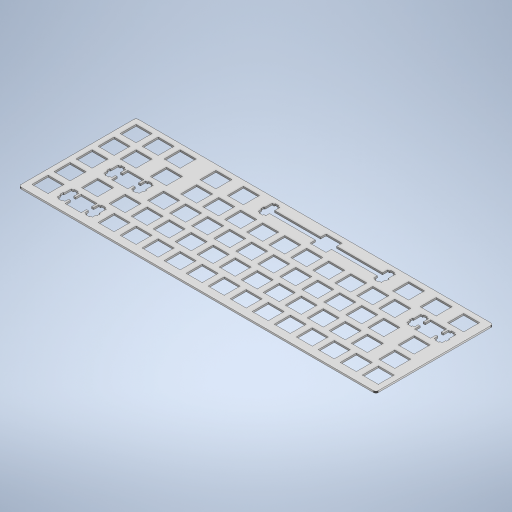
# Autodesk Inventor part: case_plate
Saved by Autodesk Inventor 2024 (Build 280153000, 153)
## iProperties
Created: 2023-08-02
Part Number: case_plate
Material: Generic
Document SubType Name: Modeling
Designer: Mika
Density: 1 g/cm^3
Appearance: Default
Author: Mika
Autodesk Inventor part; units mm, degrees
ref_plane "YZ Plane" through (0, 0, 0) normal (1, 0, 0) x (0, 1, 0)
ref_plane "XZ Plane" through (0, 0, 0) normal (0, 1, 0) x (-1, 0, 0)
ref_plane "XY Plane" through (0, 0, 0) normal (0, 0, 1) x (1, 0, 0)
sketch "Sketch1" plane through (0, 0, 0) normal (0, 1, 0) x (-1, 0, 0)
  line L0 (307.046, 101.8404) -> (307.202, 101.8337)
  line L1 (307.202, 101.8337) -> (307.359, 101.8157)
  line L2 (307.359, 101.8157) -> (307.512, 101.7853)
  line L3 (307.512, 101.7853) -> (307.665, 101.7426)
  line L4 (307.665, 101.7426) -> (307.811, 101.6876)
  line L5 (307.811, 101.6876) -> (307.953, 101.6227)
  line L6 (307.953, 101.6227) -> (308.091, 101.5458)
  line L7 (308.091, 101.5458) -> (308.222, 101.4587)
  line L8 (308.222, 101.4587) -> (308.344, 101.3609)
  line L9 (308.344, 101.3609) -> (308.46, 101.2548)
  line L10 (308.46, 101.2548) -> (308.566, 101.139)
  line L11 (308.566, 101.139) -> (308.664, 101.0166)
  line L12 (308.664, 101.0166) -> (308.751, 100.8854)
  line L13 (308.751, 100.8854) -> (308.828, 100.7478)
  line L14 (308.828, 100.7478) -> (308.894, 100.6056)
  line L15 (308.894, 100.6056) -> (308.948, 100.4596)
  line L16 (308.948, 100.4596) -> (308.991, 100.3068)
  line L17 (308.991, 100.3068) -> (309.021, 100.1537)
  line L18 (309.021, 100.1537) -> (309.039, 99.9967)
  line L19 (309.039, 99.9967) -> (309.047, 99.8398)
  line L20 (309.047, 99.8398) -> (309.047, 2.3399)
  line L21 (309.047, 2.3399) -> (309.039, 2.1842)
  line L22 (309.039, 2.1842) -> (309.021, 2.0271)
  line L23 (309.021, 2.0271) -> (308.991, 1.8741)
  line L24 (308.991, 1.8741) -> (308.948, 1.7212)
  line L25 (308.948, 1.7212) -> (308.894, 1.5751)
  line L26 (308.894, 1.5751) -> (308.828, 1.4332)
  line L27 (308.828, 1.4332) -> (308.751, 1.2954)
  line L28 (308.751, 1.2954) -> (308.664, 1.1644)
  line L29 (308.664, 1.1644) -> (308.566, 1.0418)
  line L30 (308.566, 1.0418) -> (308.46, 0.926)
  line L31 (308.46, 0.926) -> (308.344, 0.8199)
  line L32 (308.344, 0.8199) -> (308.222, 0.7221)
  line L33 (308.222, 0.7221) -> (308.091, 0.6353)
  line L34 (308.091, 0.6353) -> (307.953, 0.5581)
  line L35 (307.953, 0.5581) -> (307.811, 0.492)
  line L36 (307.811, 0.492) -> (307.665, 0.4382)
  line L37 (307.665, 0.4382) -> (307.512, 0.3955)
  line L38 (307.512, 0.3955) -> (307.359, 0.3652)
  line L39 (307.359, 0.3652) -> (307.202, 0.3473)
  line L40 (307.202, 0.3473) -> (307.045, 0.3404)
  line L41 (307.045, 0.3404) -> (2.096, 0.339)
  line L42 (2.096, 0.339) -> (1.9389, 0.3473)
  line L43 (1.9389, 0.3473) -> (1.7818, 0.3652)
  line L44 (1.7818, 0.3652) -> (1.6288, 0.3955)
  line L45 (1.6288, 0.3955) -> (1.4759, 0.4382)
  line L46 (1.4759, 0.4382) -> (1.3298, 0.492)
  line L47 (1.3298, 0.492) -> (1.1879, 0.5581)
  line L48 (1.1879, 0.5581) -> (1.0501, 0.6353)
  line L49 (1.0501, 0.6353) -> (0.9192, 0.7221)
  line L50 (0.9192, 0.7221) -> (0.7965, 0.8199)
  line L51 (0.7965, 0.8199) -> (0.6808, 0.926)
  line L52 (0.6808, 0.926) -> (0.5746, 1.0418)
  line L53 (0.5746, 1.0418) -> (0.4768, 1.1644)
  line L54 (0.4768, 1.1644) -> (0.39, 1.2954)
  line L55 (0.39, 1.2954) -> (0.3128, 1.4332)
  line L56 (0.3128, 1.4332) -> (0.248, 1.5751)
  line L57 (0.248, 1.5751) -> (0.1929, 1.7212)
  line L58 (0.1929, 1.7212) -> (0.1502, 1.8741)
  line L59 (0.1502, 1.8741) -> (0.1199, 2.0271)
  line L60 (0.1199, 2.0271) -> (0.102, 2.1842)
  line L61 (0.102, 2.1842) -> (0.0951, 2.3399)
  line L62 (0.0951, 2.3399) -> (0.0951, 99.8384)
  line L63 (0.0951, 99.8384) -> (0.102, 99.9953)
  line L64 (0.102, 99.9953) -> (0.1199, 100.1523)
  line L65 (0.1199, 100.1523) -> (0.1502, 100.3054)
  line L66 (0.1502, 100.3054) -> (0.1929, 100.4582)
  line L67 (0.1929, 100.4582) -> (0.248, 100.6042)
  line L68 (0.248, 100.6042) -> (0.3128, 100.7464)
  line L69 (0.3128, 100.7464) -> (0.39, 100.884)
  line L70 (0.39, 100.884) -> (0.4768, 101.0152)
  line L71 (0.4768, 101.0152) -> (0.5746, 101.1376)
  line L72 (0.5746, 101.1376) -> (0.6807, 101.2534)
  line L73 (0.6807, 101.2534) -> (0.7965, 101.3595)
  line L74 (0.7965, 101.3595) -> (0.9191, 101.4573)
  line L75 (0.9191, 101.4573) -> (1.0501, 101.5444)
  line L76 (1.0501, 101.5444) -> (1.1879, 101.6213)
  line L77 (1.1879, 101.6213) -> (1.3298, 101.6862)
  line L78 (1.3298, 101.6862) -> (1.4759, 101.7412)
  line L79 (1.4759, 101.7412) -> (1.6288, 101.7839)
  line L80 (1.6288, 101.7839) -> (1.7818, 101.8143)
  line L81 (1.7818, 101.8143) -> (1.9389, 101.8323)
  line L82 (1.9389, 101.8323) -> (2.096, 101.839)
  line L83 (2.096, 101.839) -> (307.046, 101.8404)
  line L84 (126.213, 18.8654) -> (126.213, 14.1663)
  line L85 (126.213, 14.1663) -> (86.4387, 14.1663)
  line L86 (86.4387, 14.1663) -> (86.4387, 17.395)
  line L87 (86.4387, 17.395) -> (84.7136, 17.395)
  line L88 (84.7136, 17.395) -> (84.7136, 18.3155)
  line L89 (84.7136, 18.3155) -> (81.5633, 18.3155)
  line L90 (81.5633, 18.3155) -> (81.5633, 17.395)
  line L91 (81.5633, 17.395) -> (79.8382, 17.395)
  line L92 (79.8382, 17.395) -> (79.8382, 14.1663)
  line L93 (79.8382, 14.1663) -> (79.0141, 14.1663)
  line L94 (79.0141, 14.1663) -> (79.0141, 11.5163)
  line L95 (79.0141, 11.5163) -> (79.8382, 11.5163)
  line L96 (79.8382, 11.5163) -> (79.8382, 5.2462)
  line L97 (79.8382, 5.2462) -> (81.5633, 5.2462)
  line L98 (81.5633, 5.2462) -> (81.5633, 4.265)
  line L99 (81.5633, 4.265) -> (84.7136, 4.265)
  line L100 (84.7136, 4.265) -> (84.7136, 5.2462)
  line L101 (84.7136, 5.2462) -> (86.4387, 5.2462)
  line L102 (86.4387, 5.2462) -> (86.4387, 9.7166)
  line L103 (86.4387, 9.7166) -> (126.213, 9.7166)
  line L104 (126.213, 9.7166) -> (126.213, 5.0161)
  line L105 (126.213, 5.0161) -> (140.064, 5.0161)
  line L106 (140.064, 5.0161) -> (140.064, 9.7166)
  line L107 (140.064, 9.7166) -> (179.838, 9.7166)
  line L108 (179.838, 9.7166) -> (179.838, 5.2462)
  line L109 (179.838, 5.2462) -> (181.563, 5.2462)
  line L110 (181.563, 5.2462) -> (181.563, 4.265)
  line L111 (181.563, 4.265) -> (184.714, 4.265)
  line L112 (184.714, 4.265) -> (184.714, 5.2462)
  line L113 (184.714, 5.2462) -> (186.439, 5.2462)
  line L114 (186.439, 5.2462) -> (186.439, 11.5163)
  line L115 (186.439, 11.5163) -> (187.263, 11.5163)
  line L116 (187.263, 11.5163) -> (187.263, 14.1663)
  line L117 (187.263, 14.1663) -> (186.439, 14.1663)
  line L118 (186.439, 14.1663) -> (186.439, 17.395)
  line L119 (186.439, 17.395) -> (184.714, 17.395)
  line L120 (184.714, 17.395) -> (184.714, 18.3155)
  line L121 (184.714, 18.3155) -> (181.563, 18.3155)
  line L122 (181.563, 18.3155) -> (181.563, 17.395)
  line L123 (181.563, 17.395) -> (179.838, 17.395)
  line L124 (179.838, 17.395) -> (179.838, 14.1663)
  line L125 (179.838, 14.1663) -> (140.064, 14.1663)
  line L126 (140.064, 14.1663) -> (140.064, 18.8654)
  line L127 (140.064, 18.8654) -> (126.213, 18.8654)
  line L128 (7.152, 18.8654) -> (21.0013, 18.8654)
  line L129 (21.0013, 18.8654) -> (21.0013, 5.0161)
  line L130 (21.0013, 5.0161) -> (7.152, 5.0161)
  line L131 (7.152, 5.0161) -> (7.152, 18.8654)
  line L132 (30.9631, 18.8654) -> (44.8137, 18.8654)
  line L133 (44.8137, 18.8654) -> (44.8137, 5.0161)
  line L134 (44.8137, 5.0161) -> (30.9631, 5.0161)
  line L135 (30.9631, 5.0161) -> (30.9631, 18.8654)
  line L136 (54.7769, 18.8654) -> (68.6262, 18.8654)
  line L137 (68.6262, 18.8654) -> (68.6262, 5.0161)
  line L138 (68.6262, 5.0161) -> (54.7769, 5.0161)
  line L139 (54.7769, 5.0161) -> (54.7769, 18.8654)
  line L140 (197.652, 18.8654) -> (211.501, 18.8654)
  line L141 (211.501, 18.8654) -> (211.501, 5.0161)
  line L142 (211.501, 5.0161) -> (197.652, 5.0161)
  line L143 (197.652, 5.0161) -> (197.652, 18.8654)
  line L144 (221.463, 18.8654) -> (235.314, 18.8654)
  line L145 (235.314, 18.8654) -> (235.314, 5.0161)
  line L146 (235.314, 5.0161) -> (221.463, 5.0161)
  line L147 (221.463, 5.0161) -> (221.463, 18.8654)
  line L148 (252.421, 18.8654) -> (266.27, 18.8654)
  line L149 (266.27, 18.8654) -> (266.27, 5.0161)
  line L150 (266.27, 5.0161) -> (252.421, 5.0161)
  line L151 (252.421, 5.0161) -> (252.421, 18.8654)
  line L152 (271.471, 18.8654) -> (285.32, 18.8654)
  line L153 (285.32, 18.8654) -> (285.32, 5.0161)
  line L154 (285.32, 5.0161) -> (271.471, 5.0161)
  line L155 (271.471, 5.0161) -> (271.471, 18.8654)
  line L156 (290.521, 18.8654) -> (304.37, 18.8654)
  line L157 (304.37, 18.8654) -> (304.37, 5.0161)
  line L158 (304.37, 5.0161) -> (290.521, 5.0161)
  line L159 (290.521, 5.0161) -> (290.521, 18.8654)
  line L160 (16.677, 37.9155) -> (16.677, 33.2163)
  line L161 (16.677, 33.2163) -> (15.0013, 33.2163)
  line L162 (15.0013, 33.2163) -> (15.0013, 36.4451)
  line L163 (15.0013, 36.4451) -> (13.276, 36.4451)
  line L164 (13.276, 36.4451) -> (13.276, 37.3655)
  line L165 (13.276, 37.3655) -> (10.1258, 37.3655)
  line L166 (10.1258, 37.3655) -> (10.1258, 36.4451)
  line L167 (10.1258, 36.4451) -> (8.4019, 36.4451)
  line L168 (8.4019, 36.4451) -> (8.4019, 33.2163)
  line L169 (8.4019, 33.2163) -> (7.5765, 33.2163)
  line L170 (7.5765, 33.2163) -> (7.5765, 30.5663)
  line L171 (7.5765, 30.5663) -> (8.4019, 30.5663)
  line L172 (8.4019, 30.5663) -> (8.4019, 24.2962)
  line L173 (8.4019, 24.2962) -> (10.1258, 24.2962)
  line L174 (10.1258, 24.2962) -> (10.1258, 23.315)
  line L175 (10.1258, 23.315) -> (13.276, 23.315)
  line L176 (13.276, 23.315) -> (13.276, 24.2962)
  line L177 (13.276, 24.2962) -> (15.0013, 24.2962)
  line L178 (15.0013, 24.2962) -> (15.0013, 28.7652)
  line L179 (15.0013, 28.7652) -> (16.677, 28.7652)
  line L180 (16.677, 28.7652) -> (16.677, 24.0661)
  line L181 (16.677, 24.0661) -> (30.5263, 24.0661)
  line L182 (30.5263, 24.0661) -> (30.5263, 28.7652)
  line L183 (30.5263, 28.7652) -> (32.202, 28.7652)
  line L184 (32.202, 28.7652) -> (32.202, 24.2962)
  line L185 (32.202, 24.2962) -> (33.9259, 24.2962)
  line L186 (33.9259, 24.2962) -> (33.9259, 23.315)
  line L187 (33.9259, 23.315) -> (37.0762, 23.315)
  line L188 (37.0762, 23.315) -> (37.0762, 24.2962)
  line L189 (37.0762, 24.2962) -> (38.8013, 24.2962)
  line L190 (38.8013, 24.2962) -> (38.8013, 30.5663)
  line L191 (38.8013, 30.5663) -> (39.6268, 30.5663)
  line L192 (39.6268, 30.5663) -> (39.6268, 33.2163)
  line L193 (39.6268, 33.2163) -> (38.8013, 33.2163)
  line L194 (38.8013, 33.2163) -> (38.8013, 36.4451)
  line L195 (38.8013, 36.4451) -> (37.0762, 36.4451)
  line L196 (37.0762, 36.4451) -> (37.0762, 37.3655)
  line L197 (37.0762, 37.3655) -> (33.9259, 37.3655)
  line L198 (33.9259, 37.3655) -> (33.9259, 36.4451)
  line L199 (33.9259, 36.4451) -> (32.202, 36.4451)
  line L200 (32.202, 36.4451) -> (32.202, 33.2163)
  line L201 (32.202, 33.2163) -> (30.5263, 33.2163)
  line L202 (30.5263, 33.2163) -> (30.5263, 37.9155)
  line L203 (30.5263, 37.9155) -> (16.677, 37.9155)
  line L204 (47.6321, 37.9155) -> (61.4825, 37.9155)
  line L205 (61.4825, 37.9155) -> (61.4825, 24.0661)
  line L206 (61.4825, 24.0661) -> (47.6321, 24.0661)
  line L207 (47.6321, 24.0661) -> (47.6321, 37.9155)
  line L208 (66.6821, 37.9155) -> (80.5325, 37.9155)
  line L209 (80.5325, 37.9155) -> (80.5325, 24.0661)
  line L210 (80.5325, 24.0661) -> (66.6821, 24.0661)
  line L211 (66.6821, 24.0661) -> (66.6821, 37.9155)
  line L212 (85.7321, 37.9155) -> (99.5825, 37.9155)
  line L213 (99.5825, 37.9155) -> (99.5825, 24.0661)
  line L214 (99.5825, 24.0661) -> (85.7321, 24.0661)
  line L215 (85.7321, 24.0661) -> (85.7321, 37.9155)
  line L216 (104.782, 37.9155) -> (118.632, 37.9155)
  line L217 (118.632, 37.9155) -> (118.632, 24.0661)
  line L218 (118.632, 24.0661) -> (104.782, 24.0661)
  line L219 (104.782, 24.0661) -> (104.782, 37.9155)
  line L220 (123.832, 37.9155) -> (137.682, 37.9155)
  line L221 (137.682, 37.9155) -> (137.682, 24.0661)
  line L222 (137.682, 24.0661) -> (123.832, 24.0661)
  line L223 (123.832, 24.0661) -> (123.832, 37.9155)
  line L224 (142.882, 37.9155) -> (156.732, 37.9155)
  line L225 (156.732, 37.9155) -> (156.732, 24.0661)
  line L226 (156.732, 24.0661) -> (142.882, 24.0661)
  line L227 (142.882, 24.0661) -> (142.882, 37.9155)
  line L228 (161.932, 37.9155) -> (175.782, 37.9155)
  line L229 (175.782, 37.9155) -> (175.782, 24.0661)
  line L230 (175.782, 24.0661) -> (161.932, 24.0661)
  line L231 (161.932, 24.0661) -> (161.932, 37.9155)
  line L232 (180.982, 37.9155) -> (194.832, 37.9155)
  line L233 (194.832, 37.9155) -> (194.832, 24.0661)
  line L234 (194.832, 24.0661) -> (180.982, 24.0661)
  line L235 (180.982, 24.0661) -> (180.982, 37.9155)
  line L236 (200.032, 37.9155) -> (213.882, 37.9155)
  line L237 (213.882, 37.9155) -> (213.882, 24.0661)
  line L238 (213.882, 24.0661) -> (200.032, 24.0661)
  line L239 (200.032, 24.0661) -> (200.032, 37.9155)
  line L240 (219.082, 37.9155) -> (232.932, 37.9155)
  line L241 (232.932, 37.9155) -> (232.932, 24.0661)
  line L242 (232.932, 24.0661) -> (219.082, 24.0661)
  line L243 (219.082, 24.0661) -> (219.082, 37.9155)
  line L244 (245.277, 37.9155) -> (259.126, 37.9155)
  line L245 (259.126, 37.9155) -> (259.126, 24.0661)
  line L246 (259.126, 24.0661) -> (245.277, 24.0661)
  line L247 (245.277, 24.0661) -> (245.277, 37.9155)
  line L248 (271.471, 37.9155) -> (285.32, 37.9155)
  line L249 (285.32, 37.9155) -> (285.32, 24.0661)
  line L250 (285.32, 24.0661) -> (271.471, 24.0661)
  line L251 (271.471, 24.0661) -> (271.471, 37.9155)
  line L252 (290.521, 37.9155) -> (304.37, 37.9155)
  line L253 (304.37, 37.9155) -> (304.37, 24.0661)
  line L254 (304.37, 24.0661) -> (290.521, 24.0661)
  line L255 (290.521, 24.0661) -> (290.521, 37.9155)
  line L256 (259.563, 56.9655) -> (259.563, 52.2661)
  line L257 (259.563, 52.2661) -> (257.889, 52.2661)
  line L258 (257.889, 52.2661) -> (257.889, 55.4951)
  line L259 (257.889, 55.4951) -> (256.162, 55.4951)
  line L260 (256.162, 55.4951) -> (256.162, 56.4155)
  line L261 (256.162, 56.4155) -> (253.013, 56.4155)
  line L262 (253.013, 56.4155) -> (253.013, 55.4951)
  line L263 (253.013, 55.4951) -> (251.288, 55.4951)
  line L264 (251.288, 55.4951) -> (251.288, 52.2661)
  line L265 (251.288, 52.2661) -> (250.464, 52.2661)
  line L266 (250.464, 52.2661) -> (250.464, 49.6164)
  line L267 (250.464, 49.6164) -> (251.288, 49.6164)
  line L268 (251.288, 49.6164) -> (251.288, 43.3462)
  line L269 (251.288, 43.3462) -> (253.013, 43.3462)
  line L270 (253.013, 43.3462) -> (253.013, 42.3651)
  line L271 (253.013, 42.3651) -> (256.162, 42.3651)
  line L272 (256.162, 42.3651) -> (256.162, 43.3462)
  line L273 (256.162, 43.3462) -> (257.889, 43.3462)
  line L274 (257.889, 43.3462) -> (257.889, 47.8151)
  line L275 (257.889, 47.8151) -> (259.563, 47.8151)
  line L276 (259.563, 47.8151) -> (259.563, 43.1161)
  line L277 (259.563, 43.1161) -> (273.414, 43.1161)
  line L278 (273.414, 43.1161) -> (273.414, 47.8151)
  line L279 (273.414, 47.8151) -> (275.088, 47.8151)
  line L280 (275.088, 47.8151) -> (275.088, 43.3462)
  line L281 (275.088, 43.3462) -> (276.813, 43.3462)
  line L282 (276.813, 43.3462) -> (276.813, 42.3651)
  line L283 (276.813, 42.3651) -> (279.964, 42.3651)
  line L284 (279.964, 42.3651) -> (279.964, 43.3462)
  line L285 (279.964, 43.3462) -> (281.689, 43.3462)
  line L286 (281.689, 43.3462) -> (281.689, 49.6164)
  line L287 (281.689, 49.6164) -> (282.513, 49.6164)
  line L288 (282.513, 49.6164) -> (282.513, 52.2661)
  line L289 (282.513, 52.2661) -> (281.689, 52.2661)
  line L290 (281.689, 52.2661) -> (281.689, 55.4951)
  line L291 (281.689, 55.4951) -> (279.964, 55.4951)
  line L292 (279.964, 55.4951) -> (279.964, 56.4155)
  line L293 (279.964, 56.4155) -> (276.813, 56.4155)
  line L294 (276.813, 56.4155) -> (276.813, 55.4951)
  line L295 (276.813, 55.4951) -> (275.088, 55.4951)
  line L296 (275.088, 55.4951) -> (275.088, 52.2661)
  line L297 (275.088, 52.2661) -> (273.414, 52.2661)
  line L298 (273.414, 52.2661) -> (273.414, 56.9655)
  line L299 (273.414, 56.9655) -> (259.563, 56.9655)
  line L300 (11.9131, 56.9655) -> (25.7638, 56.9655)
  line L301 (25.7638, 56.9655) -> (25.7638, 43.1161)
  line L302 (25.7638, 43.1161) -> (11.9131, 43.1161)
  line L303 (11.9131, 43.1161) -> (11.9131, 56.9655)
  line L304 (38.1071, 56.9655) -> (51.9575, 56.9655)
  line L305 (51.9575, 56.9655) -> (51.9575, 43.1161)
  line L306 (51.9575, 43.1161) -> (38.1071, 43.1161)
  line L307 (38.1071, 43.1161) -> (38.1071, 56.9655)
  line L308 (57.1571, 56.9655) -> (71.0075, 56.9655)
  line L309 (71.0075, 56.9655) -> (71.0075, 43.1161)
  line L310 (71.0075, 43.1161) -> (57.1571, 43.1161)
  line L311 (57.1571, 43.1161) -> (57.1571, 56.9655)
  line L312 (76.2071, 56.9655) -> (90.0575, 56.9655)
  line L313 (90.0575, 56.9655) -> (90.0575, 43.1161)
  line L314 (90.0575, 43.1161) -> (76.2071, 43.1161)
  line L315 (76.2071, 43.1161) -> (76.2071, 56.9655)
  line L316 (95.2571, 56.9655) -> (109.107, 56.9655)
  line L317 (109.107, 56.9655) -> (109.107, 43.1161)
  line L318 (109.107, 43.1161) -> (95.2571, 43.1161)
  line L319 (95.2571, 43.1161) -> (95.2571, 56.9655)
  line L320 (114.307, 56.9655) -> (128.157, 56.9655)
  line L321 (128.157, 56.9655) -> (128.157, 43.1161)
  line L322 (128.157, 43.1161) -> (114.307, 43.1161)
  line L323 (114.307, 43.1161) -> (114.307, 56.9655)
  line L324 (133.357, 56.9655) -> (147.207, 56.9655)
  line L325 (147.207, 56.9655) -> (147.207, 43.1161)
  line L326 (147.207, 43.1161) -> (133.357, 43.1161)
  line L327 (133.357, 43.1161) -> (133.357, 56.9655)
  line L328 (152.407, 56.9655) -> (166.257, 56.9655)
  line L329 (166.257, 56.9655) -> (166.257, 43.1161)
  line L330 (166.257, 43.1161) -> (152.407, 43.1161)
  line L331 (152.407, 43.1161) -> (152.407, 56.9655)
  line L332 (171.457, 56.9655) -> (185.307, 56.9655)
  line L333 (185.307, 56.9655) -> (185.307, 43.1161)
  line L334 (185.307, 43.1161) -> (171.457, 43.1161)
  line L335 (171.457, 43.1161) -> (171.457, 56.9655)
  line L336 (190.507, 56.9655) -> (204.357, 56.9655)
  line L337 (204.357, 56.9655) -> (204.357, 43.1161)
  line L338 (204.357, 43.1161) -> (190.507, 43.1161)
  line L339 (190.507, 43.1161) -> (190.507, 56.9655)
  line L340 (209.557, 56.9655) -> (223.407, 56.9655)
  line L341 (223.407, 56.9655) -> (223.407, 43.1161)
  line L342 (223.407, 43.1161) -> (209.557, 43.1161)
  line L343 (209.557, 43.1161) -> (209.557, 56.9655)
  line L344 (228.607, 56.9655) -> (242.457, 56.9655)
  line L345 (242.457, 56.9655) -> (242.457, 43.1161)
  line L346 (242.457, 43.1161) -> (228.607, 43.1161)
  line L347 (228.607, 43.1161) -> (228.607, 56.9655)
  line L348 (290.521, 56.9655) -> (304.37, 56.9655)
  line L349 (304.37, 56.9655) -> (304.37, 43.1161)
  line L350 (304.37, 43.1161) -> (290.521, 43.1161)
  line L351 (290.521, 43.1161) -> (290.521, 56.9655)
  line L352 (9.5319, 76.0155) -> (23.3826, 76.0155)
  line L353 (23.3826, 76.0155) -> (23.3826, 62.1661)
  line L354 (23.3826, 62.1661) -> (9.5319, 62.1661)
  line L355 (9.5319, 62.1661) -> (9.5319, 76.0155)
  line L356 (33.3458, 76.0155) -> (47.195, 76.0155)
  line L357 (47.195, 76.0155) -> (47.195, 62.1661)
  line L358 (47.195, 62.1661) -> (33.3458, 62.1661)
  line L359 (33.3458, 62.1661) -> (33.3458, 76.0155)
  line L360 (52.3956, 76.0155) -> (66.245, 76.0155)
  line L361 (66.245, 76.0155) -> (66.245, 62.1661)
  line L362 (66.245, 62.1661) -> (52.3956, 62.1661)
  line L363 (52.3956, 62.1661) -> (52.3956, 76.0155)
  line L364 (71.4456, 76.0155) -> (85.295, 76.0155)
  line L365 (85.295, 76.0155) -> (85.295, 62.1661)
  line L366 (85.295, 62.1661) -> (71.4456, 62.1661)
  line L367 (71.4456, 62.1661) -> (71.4456, 76.0155)
  line L368 (90.4946, 76.0155) -> (104.345, 76.0155)
  line L369 (104.345, 76.0155) -> (104.345, 62.1661)
  line L370 (104.345, 62.1661) -> (90.4946, 62.1661)
  line L371 (90.4946, 62.1661) -> (90.4946, 76.0155)
  line L372 (109.545, 76.0155) -> (123.395, 76.0155)
  line L373 (123.395, 76.0155) -> (123.395, 62.1661)
  line L374 (123.395, 62.1661) -> (109.545, 62.1661)
  line L375 (109.545, 62.1661) -> (109.545, 76.0155)
  line L376 (128.595, 76.0155) -> (142.445, 76.0155)
  line L377 (142.445, 76.0155) -> (142.445, 62.1661)
  line L378 (142.445, 62.1661) -> (128.595, 62.1661)
  line L379 (128.595, 62.1661) -> (128.595, 76.0155)
  line L380 (147.645, 76.0155) -> (161.495, 76.0155)
  line L381 (161.495, 76.0155) -> (161.495, 62.1661)
  line L382 (161.495, 62.1661) -> (147.645, 62.1661)
  line L383 (147.645, 62.1661) -> (147.645, 76.0155)
  line L384 (166.696, 76.0155) -> (180.545, 76.0155)
  line L385 (180.545, 76.0155) -> (180.545, 62.1661)
  line L386 (180.545, 62.1661) -> (166.696, 62.1661)
  line L387 (166.696, 62.1661) -> (166.696, 76.0155)
  line L388 (185.746, 76.0155) -> (199.595, 76.0155)
  line L389 (199.595, 76.0155) -> (199.595, 62.1661)
  line L390 (199.595, 62.1661) -> (185.746, 62.1661)
  line L391 (185.746, 62.1661) -> (185.746, 76.0155)
  line L392 (204.796, 76.0155) -> (218.645, 76.0155)
  line L393 (218.645, 76.0155) -> (218.645, 62.1661)
  line L394 (218.645, 62.1661) -> (204.796, 62.1661)
  line L395 (204.796, 62.1661) -> (204.796, 76.0155)
  line L396 (223.846, 76.0155) -> (237.695, 76.0155)
  line L397 (237.695, 76.0155) -> (237.695, 62.1661)
  line L398 (237.695, 62.1661) -> (223.846, 62.1661)
  line L399 (223.846, 62.1661) -> (223.846, 76.0155)
  line L400 (242.896, 76.0155) -> (256.745, 76.0155)
  line L401 (256.745, 76.0155) -> (256.745, 62.1661)
  line L402 (256.745, 62.1661) -> (242.896, 62.1661)
  line L403 (242.896, 62.1661) -> (242.896, 76.0155)
  line L404 (266.707, 76.0155) -> (280.557, 76.0155)
  line L405 (280.557, 76.0155) -> (280.557, 62.1661)
  line L406 (280.557, 62.1661) -> (266.707, 62.1661)
  line L407 (266.707, 62.1661) -> (266.707, 76.0155)
  line L408 (290.521, 76.0155) -> (304.37, 76.0155)
  line L409 (304.37, 76.0155) -> (304.37, 62.1661)
  line L410 (304.37, 62.1661) -> (290.521, 62.1661)
  line L411 (290.521, 62.1661) -> (290.521, 76.0155)
  line L412 (261.946, 95.0655) -> (261.946, 90.3661)
  line L413 (261.946, 90.3661) -> (260.27, 90.3661)
  line L414 (260.27, 90.3661) -> (260.27, 93.5951)
  line L415 (260.27, 93.5951) -> (258.546, 93.5951)
  line L416 (258.546, 93.5951) -> (258.546, 94.5155)
  line L417 (258.546, 94.5155) -> (255.396, 94.5155)
  line L418 (255.396, 94.5155) -> (255.396, 93.5951)
  line L419 (255.396, 93.5951) -> (253.67, 93.5951)
  line L420 (253.67, 93.5951) -> (253.67, 90.3661)
  line L421 (253.67, 90.3661) -> (252.845, 90.3661)
  line L422 (252.845, 90.3661) -> (252.845, 87.7164)
  line L423 (252.845, 87.7164) -> (253.67, 87.7164)
  line L424 (253.67, 87.7164) -> (253.67, 81.4462)
  line L425 (253.67, 81.4462) -> (255.396, 81.4462)
  line L426 (255.396, 81.4462) -> (255.396, 80.4651)
  line L427 (255.396, 80.4651) -> (258.546, 80.4651)
  line L428 (258.546, 80.4651) -> (258.546, 81.4462)
  line L429 (258.546, 81.4462) -> (260.27, 81.4462)
  line L430 (260.27, 81.4462) -> (260.27, 85.9151)
  line L431 (260.27, 85.9151) -> (261.946, 85.9151)
  line L432 (261.946, 85.9151) -> (261.946, 81.2161)
  line L433 (261.946, 81.2161) -> (275.795, 81.2161)
  line L434 (275.795, 81.2161) -> (275.795, 85.9151)
  line L435 (275.795, 85.9151) -> (277.471, 85.9151)
  line L436 (277.471, 85.9151) -> (277.471, 81.4462)
  line L437 (277.471, 81.4462) -> (279.196, 81.4462)
  line L438 (279.196, 81.4462) -> (279.196, 80.4651)
  line L439 (279.196, 80.4651) -> (282.345, 80.4651)
  line L440 (282.345, 80.4651) -> (282.345, 81.4462)
  line L441 (282.345, 81.4462) -> (284.07, 81.4462)
  line L442 (284.07, 81.4462) -> (284.07, 87.7164)
  line L443 (284.07, 87.7164) -> (284.896, 87.7164)
  line L444 (284.896, 87.7164) -> (284.896, 90.3661)
  line L445 (284.896, 90.3661) -> (284.07, 90.3661)
  line L446 (284.07, 90.3661) -> (284.07, 93.5951)
  line L447 (284.07, 93.5951) -> (282.345, 93.5951)
  line L448 (282.345, 93.5951) -> (282.345, 94.5155)
  line L449 (282.345, 94.5155) -> (279.196, 94.5155)
  line L450 (279.196, 94.5155) -> (279.196, 93.5951)
  line L451 (279.196, 93.5951) -> (277.471, 93.5951)
  line L452 (277.471, 93.5951) -> (277.471, 90.3661)
  line L453 (277.471, 90.3661) -> (275.795, 90.3661)
  line L454 (275.795, 90.3661) -> (275.795, 95.0655)
  line L455 (275.795, 95.0655) -> (261.946, 95.0655)
  line L456 (4.7708, 95.0655) -> (18.6201, 95.0655)
  line L457 (18.6201, 95.0655) -> (18.6201, 81.2161)
  line L458 (18.6201, 81.2161) -> (4.7708, 81.2161)
  line L459 (4.7708, 81.2161) -> (4.7708, 95.0655)
  line L460 (23.8208, 95.0655) -> (37.67, 95.0655)
  line L461 (37.67, 95.0655) -> (37.67, 81.2161)
  line L462 (37.67, 81.2161) -> (23.8208, 81.2161)
  line L463 (23.8208, 81.2161) -> (23.8208, 95.0655)
  line L464 (42.8706, 95.0655) -> (56.72, 95.0655)
  line L465 (56.72, 95.0655) -> (56.72, 81.2161)
  line L466 (56.72, 81.2161) -> (42.8706, 81.2161)
  line L467 (42.8706, 81.2161) -> (42.8706, 95.0655)
  line L468 (61.9206, 95.0655) -> (75.77, 95.0655)
  line L469 (75.77, 95.0655) -> (75.77, 81.2161)
  line L470 (75.77, 81.2161) -> (61.9206, 81.2161)
  line L471 (61.9206, 81.2161) -> (61.9206, 95.0655)
  line L472 (80.9706, 95.0655) -> (94.82, 95.0655)
  line L473 (94.82, 95.0655) -> (94.82, 81.2161)
  line L474 (94.82, 81.2161) -> (80.9706, 81.2161)
  line L475 (80.9706, 81.2161) -> (80.9706, 95.0655)
  line L476 (100.021, 95.0655) -> (113.87, 95.0655)
  line L477 (113.87, 95.0655) -> (113.87, 81.2161)
  line L478 (113.87, 81.2161) -> (100.021, 81.2161)
  line L479 (100.021, 81.2161) -> (100.021, 95.0655)
  line L480 (119.071, 95.0655) -> (132.92, 95.0655)
  line L481 (132.92, 95.0655) -> (132.92, 81.2161)
  line L482 (132.92, 81.2161) -> (119.071, 81.2161)
  line L483 (119.071, 81.2161) -> (119.071, 95.0655)
  line L484 (138.121, 95.0655) -> (151.97, 95.0655)
  line L485 (151.97, 95.0655) -> (151.97, 81.2161)
  line L486 (151.97, 81.2161) -> (138.121, 81.2161)
  line L487 (138.121, 81.2161) -> (138.121, 95.0655)
  line L488 (157.171, 95.0655) -> (171.02, 95.0655)
  line L489 (171.02, 95.0655) -> (171.02, 81.2161)
  line L490 (171.02, 81.2161) -> (157.171, 81.2161)
  line L491 (157.171, 81.2161) -> (157.171, 95.0655)
  line L492 (176.221, 95.0655) -> (190.07, 95.0655)
  line L493 (190.07, 95.0655) -> (190.07, 81.2161)
  line L494 (190.07, 81.2161) -> (176.221, 81.2161)
  line L495 (176.221, 81.2161) -> (176.221, 95.0655)
  line L496 (195.271, 95.0655) -> (209.12, 95.0655)
  line L497 (209.12, 95.0655) -> (209.12, 81.2161)
  line L498 (209.12, 81.2161) -> (195.271, 81.2161)
  line L499 (195.271, 81.2161) -> (195.271, 95.0655)
  line L500 (214.321, 95.0655) -> (228.17, 95.0655)
  line L501 (228.17, 95.0655) -> (228.17, 81.2161)
  line L502 (228.17, 81.2161) -> (214.321, 81.2161)
  line L503 (214.321, 81.2161) -> (214.321, 95.0655)
  line L504 (233.371, 95.0655) -> (247.22, 95.0655)
  line L505 (247.22, 95.0655) -> (247.22, 81.2161)
  line L506 (247.22, 81.2161) -> (233.371, 81.2161)
  line L507 (233.371, 81.2161) -> (233.371, 95.0655)
  line L508 (290.521, 95.0655) -> (304.37, 95.0655)
  line L509 (304.37, 95.0655) -> (304.37, 81.2161)
  line L510 (304.37, 81.2161) -> (290.521, 81.2161)
  line L511 (290.521, 81.2161) -> (290.521, 95.0655)
  point P0 (0, 0)
  point P1 (0.0951, 99.8382)
  point P2 (2.096, 0.339)
  point P3 (309.047, 2.3399)
  point P4 (309.047, 99.84)
  point P5 (4.7708, 81.2161)
  point P6 (7.152, 5.0161)
  dimension "d0" = 308.9519
  dimension "d1" = 101.5
  constraints: 1024 end point, 1 parallel
  measures "d0" distance between parallel lines of L20 L62
  measures "d1" distance between parallel lines of L83 L41
extrude "Extrusion1" add sketch "Sketch1" along normal blind 1.48
body "Solid1"
